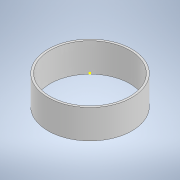
# Autodesk Inventor part: BigCollar1
Saved by Autodesk Inventor 2020 (Build 240168000, 168)
## iProperties
Created: 2020-05-10
Part Number: BigCollar1
Material: Generic
Document SubType Name: Modeling
Designer: Spencer
Density: 1 g/cm^3
Appearance: Default
Author: Spencer
## iProperties of the stored document _3DPrint.ipt
Created: 2020-05-10
Part Number: _3DPrint
Material: Generic
Document SubType Name: Modeling
Designer: Spencer
Density: 1 g/cm^3
Appearance: Default
Author: Spencer
Autodesk Inventor part; units mm, degrees
ref_plane "YZ Plane" through (0, 0, 0) normal (1, 0, 0) x (0, 1, 0)
ref_plane "XZ Plane" through (0, 0, 0) normal (0, 1, 0) x (-1, 0, 0)
ref_plane "XY Plane" through (0, 0, 0) normal (0, 0, 1) x (1, 0, 0)
sketch "Sketch1" plane through (0, 0, 0) normal (0, 1, 0) x (-1, 0, 0)
  circle A0 centre (0, 0) radius 9.65
  circle A1 centre (0, 0) radius 10.15
  dimension "d0" = 19.3
  dimension "d1" = 20.3
  constraints: 2 centre point, 2 coincident
  measures "d0" diameter of A0
  measures "d1" diameter of A1
extrude "Extrusion1" add sketch "Sketch1" along normal blind 7
sketch "Sketch2" plane through (0, 7, 0) normal (0, 1, 0) x (1, 0, 0)
  point P0 (0, 0)
body "Solid1"
